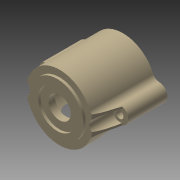
# Autodesk Inventor part: Encoder Mount Mk4
Saved by Autodesk Inventor 2013 (Build 170138000, 138)
## iProperties
Created: 2013-06-28
Part Number: Encoder Mount Mk4
Material: Generic
Document SubType Name: Modeling
Designer: mvarma
Density: 1 g/cm^3
Author: mvarma
Autodesk Inventor part; units mm, degrees
ref_plane "YZ Plane" through (0, 0, 0) normal (1, 0, 0) x (0, 1, 0)
ref_plane "XZ Plane" through (0, 0, 0) normal (0, 1, 0) x (-1, 0, 0)
ref_plane "XY Plane" through (0, 0, 0) normal (0, 0, 1) x (1, 0, 0)
sketch "Sketch1" plane through (0, 0, 0) normal (0, 0, 1) x (1, 0, 0)
  circle A0 centre (0, 0) radius 9.2075
  circle A1 centre (0, 0) radius 17.4625 construction
  circle A2 centre (0, 0) radius 12.7
  circle A3 centre (-17.4625, 0) radius 4.1275
  circle A4 centre (-17.4625, 0) radius 3.175
  line L0 (-17.4625, 0) -> (0, 0) construction
  circle A5 centre (0, 0) radius 5.3975
  line L1 (0, 0) -> (17.4625, 0) construction
  circle A6 centre (17.4625, 0) radius 3.175
  circle A7 centre (17.4625, 0) radius 4.1275
  circle A8 centre (0, 0) radius 15.875
  line L2 (-18.7325, 3.9273) -> (-18.7325, 2.9099)
  line L3 (-18.7325, 2.9099) -> (-18.7325, -2.9099)
  line L4 (-18.7325, -2.9099) -> (-18.7325, -3.9273)
  line L5 (18.7325, 3.9273) -> (18.7325, 2.9099)
  line L6 (18.7325, 2.9099) -> (18.7325, -2.9099)
  circle A9 centre (0, 0) radius 11.1125
  line L7 (18.7325, -2.9099) -> (18.7325, -3.9273)
  dimension "d0" = 18.415
  dimension "d2" = 34.925
  dimension "d3" = 25.4
  dimension "d4" = 8.255
  dimension "d5" = 6.35
  dimension "d7" = 10.795
  dimension "d12" = 6.35
  dimension "d13" = 8.255
  dimension "d16" = 31.75
  dimension "d17" = 1.27
  dimension "d18" = 1.27
  dimension "d28" = 22.225
  constraints: 22 coincident, 16 end point, 10 centre point, 10 point on circle, 3 perpendicular, 2 horizontal, 2 parallel, 1 collinear
  measures "d0" diameter of A0
  measures "d2" diameter of A1
  measures "d3" diameter of A2
  measures "d4" diameter of A3
  measures "d5" diameter of A4
  measures "d7" diameter of A5
  measures "d12" diameter of A6
  measures "d13" diameter of A7
  measures "d16" diameter of A8
  measures "d17" distance from line of A1.start L2
  measures "d18" distance from line of L5 L1.end
  measures "d28" diameter of A9
extrude "Extrusion1" add sketch "Sketch1" along normal blind 1.27 contours A2 | A9
extrude "Extrusion2" add sketch "Sketch1" against normal blind 3.175 contours A0 | A8 A7 A3 | A3 A8 A4 | A8 A6 A7 | A4 A8 | A8 A6 | A9
extrude "Extrusion3" add sketch "Sketch1" against normal blind 30.7023 contours L2 A4 L4 A3 | A3 A8 A4 L2 | L4 A4 A8 A3 | A8 A7 A3 | A3 A8 A4 | L3 A4 | A4 A8 L3 | A8 A6 A7 | A7 L5 A6 A8 | A4 A8 | A8 A6 L7 A7 | A7 L7 A6 L5 | A8 A6 | A6 L6 A8 | A6 L6
extrude "Extrusion4" cut sketch "Sketch1" against normal blind 11.6522 contours L2 A4 L4 A3 | L3 A4 | A4 A8 L3 | A4 A8 | A7 L7 A6 L5 | A8 A6 | A6 L6 A8 | A6 L6
fillet "Fillet1" radius 3.175 4 edges at (-15.4594, -3.6088, -15.3511) (-15.4594, 3.6088, -15.3511) (15.4594, -3.6088, -15.3511) (15.4594, 3.6088, -15.3511)
extrude "Extrusion5" add sketch "Sketch1" against normal up to surface (30.7023 mm away) contours A2
chamfer "Chamfer1" distance 3.175 distance2 11.6522 1 edges at (-18.7325, -3.4186, 0) measured on face at (-18.2325, -3.4186, 0)
chamfer "Chamfer2" distance 3.175 distance2 11.6522 1 edges at (-18.7325, 3.4186, 0) measured on face at (-18.2325, 3.4186, 0)
chamfer "Chamfer3" distance 3.175 distance2 11.6522 1 edges at (18.7325, -3.4186, 0) measured on face at (18.2325, -3.4186, 0)
chamfer "Chamfer4" distance 3.175 distance2 11.6522 1 edges at (18.7325, 3.4186, 0) measured on face at (18.2325, 3.4186, 0)
hole "Hole1" at (-17.4625, 0, 0) at (17.4625, 0, 0) direction (0, 0, -1) diameter 3.6576 end through all clearance for "Flat Head Machine Screw (82)" size "#6" standard "Ansi Unified Screw Threads"
sketch "Sketch2" plane through (0, 0, 0) normal (1, 0, 0) x (0, 1, 0)
  line L0 (-16.4042, -5.8261) -> (-12.1708, -5.8261)
  line L1 (-7.9375, -10.0595) -> (-7.9375, -23.8178)
  line L2 (-12.1708, -28.0511) -> (-16.4042, -28.0511)
  line L3 (-20.6375, -23.8178) -> (-20.6375, -10.0595)
  line L4 (-15.875, -30.7023) -> (-6.0844, -30.7023) projected
  line L5 (11.1125, -3.175) -> (-11.1125, -3.175) projected
  arc A0 (-16.4042, -5.8261) -> (-20.6375, -10.0595) centre (-16.4042, -10.0595) ccw
  arc A1 (-7.9375, -10.0595) -> (-12.1708, -5.8261) centre (-12.1708, -10.0595) ccw
  arc A2 (-20.6375, -23.8178) -> (-16.4042, -28.0511) centre (-16.4042, -23.8178) ccw
  arc A3 (-12.1708, -28.0511) -> (-7.9375, -23.8178) centre (-12.1708, -23.8178) ccw
  point P0 (0, 0)
  point P1 (-7.9375, -28.0511)
  point P2 (-7.9375, -5.8261)
  dimension "d44" = 2.6511
  dimension "d45" = 22.225
  dimension "d46" = 2.6511
  dimension "d47" = 12.7
  dimension "d48" = 20.6375
  dimension "d49" = 4.2333
  constraints: 8 end point, 8 point on circle, 8 tangent, 4 centre point, 4 point on line, 3 equal radius, 2 parallel, 1 horizontal, 1 perpendicular
  measures "d44" distance between parallel lines of L2 L4
  measures "d45" distance of point (-7.938, -5.826) point (-7.938, -28.051)
  measures "d46" distance between parallel lines of L0 L5
  measures "d47" distance between parallel lines of L1 L3
  measures "d48" distance from line of point (0, 0) L3
  measures "d49" radius of A0
extrude "Extrusion6" cut sketch "Sketch2" along normal through all both and the other way through all
equation "\"d44\" = d46"
body "Solid1"
